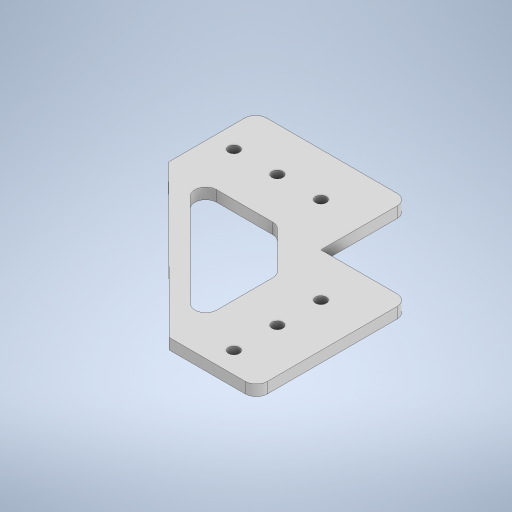
# Autodesk Inventor part: Cut L-Bracket (5x5)
Saved by Autodesk Inventor 2023 (Build 270158030, 158C)
## iProperties
Created: 2022-07-21
Part Number: Cut L-Bracket (5x5)
Material: Generic
Document SubType Name: Modeling
Designer: rm0990889
Density: 1 g/cm^3
Appearance: Default
Author: rm0990889
Autodesk Inventor part; units mm, degrees
ref_plane "YZ Plane" through (0, 0, 0) normal (1, 0, 0) x (0, 1, 0)
ref_plane "XZ Plane" through (0, 0, 0) normal (0, 1, 0) x (-1, 0, 0)
ref_plane "XY Plane" through (0, 0, 0) normal (0, 0, 1) x (1, 0, 0)
sketch "Sketch1" plane through (0, 0, 0) normal (0, 1, 0) x (-1, 0, 0)
  line L0 (28.575, 5.149) -> (50.5384, 5.149)
  line L1 (0, 33.724) -> (0, 50.8)
  line L2 (25.4, 8.324) -> (25.4, 30.549)
  line L3 (25.4, 30.549) -> (3.175, 30.549)
  arc A0 (25.4, 8.324) -> (28.575, 5.149) centre (28.575, 8.324) ccw
  arc A1 (0, 33.724) -> (3.175, 30.549) centre (3.175, 33.724) ccw
  circle A2 centre (12.7, 43.249) radius 1.5875
  circle A3 centre (38.1, 17.849) radius 1.5875
  circle A4 centre (50.8, 17.849) radius 1.5875
  circle A5 centre (63.5, 17.849) radius 1.5875
  line L4 (50.5384, 5.149) -> (66.675, 5.149)
  line L5 (69.85, 8.324) -> (69.85, 30.549)
  arc A6 (66.675, 5.149) -> (69.85, 8.324) centre (66.675, 8.324) ccw
  circle A7 centre (12.7, 55.949) radius 1.5875
  circle A8 centre (12.7, 68.649) radius 1.5875
  line L6 (0, 50.8) -> (0, 71.6223)
  line L7 (3.175, 74.7973) -> (25.4, 74.7973)
  arc A9 (3.175, 74.7973) -> (0, 71.6223) centre (3.175, 71.6223) ccw
  line L8 (25.4, 74.7973) -> (69.85, 30.549)
  line L9 (26.3299, 42.319) -> (37.1701, 31.4789)
  line L10 (39.4151, 30.549) -> (55.8349, 30.549)
  line L11 (58.0799, 35.969) -> (30.8201, 63.2289)
  line L12 (25.4, 60.9838) -> (25.4, 44.5641)
  arc A10 (30.8201, 63.2289) -> (25.4, 60.9838) centre (28.575, 60.9838) ccw
  arc A11 (55.8349, 30.549) -> (58.0799, 35.969) centre (55.8349, 33.724) ccw
  arc A12 (37.1701, 31.4789) -> (39.4151, 30.549) centre (39.4151, 33.724) ccw
  arc A13 (25.4, 44.5641) -> (26.3299, 42.319) centre (28.575, 44.5641) ccw
  point P0 (0, 0)
  point P1 (25.4, 5.149)
  point P2 (0, 42.262)
  point P3 (25.4, 19.4365)
  point P4 (39.5567, 5.149)
  point P5 (69.85, 5.149)
  point P6 (0, 74.7973)
  point P7 (14.2875, 74.7973)
  point P8 (38.1, 30.549)
  point P9 (63.5, 30.549)
  dimension "d0" = 50.8
  dimension "d1" = 50.8
  dimension "d2" = 25.4
  dimension "d3" = 3.175
  dimension "d4" = 3.175
  dimension "d5" = 12.7
  dimension "d6" = 12.7
  dimension "d7" = 3.175
  dimension "d8" = 12.7
  dimension "d9" = 12.7
  dimension "d12" = 12.7
  dimension "d17" = 25.4
  dimension "d18" = 6.35
  dimension "d19" = 3.175
  dimension "d22" = 12.7
  dimension "d27" = 25.4
  dimension "d28" = 6.35
  dimension "d29" = 3.175
  dimension "d30" = 25.4
  dimension "d31" = 6.35
  dimension "d32" = 3.175
  constraints: 26 end point, 16 point on circle, 16 tangent, 14 centre point, 10 point on line, 4 equal radius, 4 midpoint, 4 perpendicular, 4 vertical, 3 horizontal, 1 parallel, 8 other
  measures "d0" distance of point (0, 0) L0.end
  measures "d1" distance of point (0, 0) L1.end
  measures "d2" distance of point (25.4, 5.149) L2.end
  measures "d3" radius of A0
  measures "d4" diameter of A2
  measures "d5" distance from line of L3 A2.centre
  measures "d6" horizontal distance of point (0, 42.262) A2.centre
  measures "d7" diameter of A3
  measures "d8" horizontal distance of point (25.4, 19.436) A3.centre
  measures "d9" vertical distance of point (39.557, 5.149) A3.centre
  measures "d12" distance of A3.centre A4.centre
  measures "d17" distance of point (69.85, 5.149) L5.end
  measures "d18" distance from line of A5.centre L5
  measures "d19" radius of A6
  measures "d22" distance of A2.centre A7.centre
  measures "d27" distance of point (0, 74.797) L7.end
  measures "d28" distance of A8.centre point (14.287, 74.797)
  measures "d29" radius of A9
  measures "d30" distance of point (38.1, 30.549) point (63.5, 30.549)
  measures "d31" distance of point (63.5, 30.549) L5.end
  measures "d32" radius of A10
extrude "Extrusion1" add sketch "Sketch1" along normal blind 3.175
body "Solid1"
